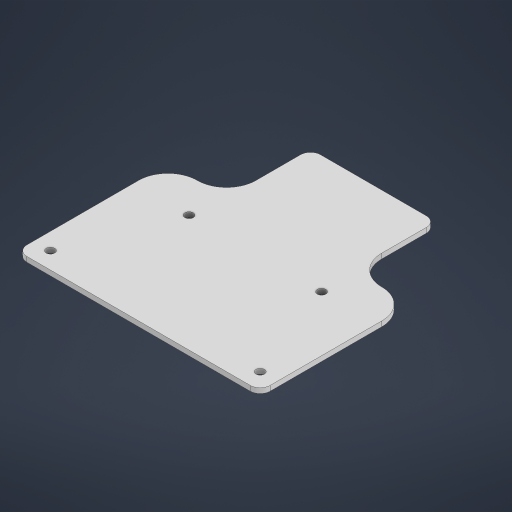
# Autodesk Inventor part: chasis_arriba
Saved by Autodesk Inventor 2023 (Build 270158000, 158)
## iProperties
Created: 2022-08-22
Part Number: chasis_arriba
Material: Generic
Document SubType Name: Modeling
Designer: marat
Density: 1 g/cm^3
Appearance: Default
Author: marat
Autodesk Inventor part; units mm, degrees
ref_plane "YZ Plane" through (0, 0, 0) normal (1, 0, 0) x (0, 1, 0)
ref_plane "XZ Plane" through (0, 0, 0) normal (0, 1, 0) x (-1, 0, 0)
ref_plane "XY Plane" through (0, 0, 0) normal (0, 0, 1) x (1, 0, 0)
sketch "Sketch1" plane through (0, 0, 0) normal (0, 1, 0) x (-1, 0, 0)
  line L0 (72.5, -45) -> (-72.5, -45)
  line L1 (-72.5, -45) -> (-72.5, 45)
  line L2 (-72.5, 45) -> (72.5, 45)
  line L3 (72.5, 45) -> (72.5, -45)
  line L4 (72.5, -45) -> (-72.5, 45) construction
  line L5 (-72.5, -45) -> (72.5, 45) construction
  point P0 (0, 0)
  dimension "d0" = 145
  dimension "d1" = 90
  constraints: 12 end point, 2 midpoint, 2 parallel, 1 horizontal, 1 perpendicular
  measures "d0" distance of L1.end L2.end
  measures "d1" distance of L0.end L1.end
extrude "Extrusion1" add sketch "Sketch1" along normal blind 3
sketch "Sketch4" plane through (72.5, 0, -45) normal (0, 0, -1) x (-1, 0, 0)
  line L0 (35, 3) -> (110, 3)
  line L1 (110, 3) -> (110, 0)
  line L2 (110, 0) -> (35, 0)
  line L3 (35, 0) -> (35, 3)
  line L4 (35, 3) -> (110, 0) construction
  line L5 (110, 3) -> (35, 0) construction
  line L6 (0, 3) -> (145, 3) projected
  point P0 (72.5, 0)
  point P1 (72.5, 1.5)
  dimension "d28" = 75
  dimension "d29" = 3
  dimension "d30" = 0
  constraints: 12 end point, 2 midpoint, 2 parallel, 1 horizontal, 1 perpendicular
  measures "d28" distance of L1.end L2.end
  measures "d29" distance of L0.end L1.end
  measures "d30" distance between parallel lines of L6 L0
extrude "Extrusion3" add sketch "Sketch4" along normal blind 50
sketch "Sketch3" plane through (0, 3, 0) normal (0, 1, 0) x (1, 0, 0)
  circle A0 centre (62.5, -34.9998) radius 2.5
  circle A1 centre (-62.5, -35) radius 2.5
  circle A2 centre (-39.5, 24.592) radius 2.5
  circle A3 centre (39.5, 24.5944) radius 2.5
  line L0 (-72.5, 45) -> (-72.5, -45) projected
  line L1 (-72.5, -45) -> (72.5, -45) projected
  point P0 (0, 0)
  dimension "d4" = 5
  dimension "d7" = 5
  dimension "d10" = 5
  dimension "d13" = 5
  dimension "d20" = 79
  dimension "d21" = 125
  dimension "d22" = 23
  dimension "d23" = 59.592
  dimension "d24" = 10
  dimension "d25" = 10
  constraints: 4 centre point
  measures "d4" diameter of A0
  measures "d7" diameter of A1
  measures "d10" diameter of A2
  measures "d13" diameter of A3
  measures "d20" distance of A3.centre A2.centre
  measures "d21" distance of A0.centre A1.centre
  measures "d22" horizontal distance of A2.centre A1.centre
  measures "d23" vertical distance of A1.centre A2.centre
  measures "d24" distance from line of L0 A1.centre
  measures "d25" distance from line of L1 A1.centre
extrude "Extrusion2" cut sketch "Sketch3" against normal through all
fillet "Fillet1" radius 6 4 edges at (72.5, 1.5, 45) (-72.5, 1.5, 45) (-37.5, 1.5, -95) (37.5, 1.5, -95)
fillet "Fillet2" radius 17.5 4 edges at (72.5, 1.5, -45) (-72.5, 1.5, -45) (37.5, 1.5, -45) (-37.5, 1.5, -45)
body "Solid1"
